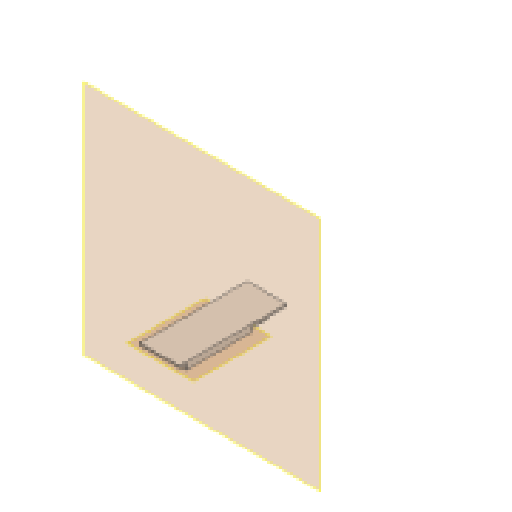
# Autodesk Inventor part: MCU seatbelt
Saved by Autodesk Inventor 2023 (Build 270158000, 158)
## iProperties
Created: 2025-01-03
Part Number: MCU seatbelt
Material: Generic
Document SubType Name: Modeling
Designer: jonwo
Density: 1 g/cm^3
Appearance: Default
Author: jonwo
Autodesk Inventor part; units mm, degrees
ref_plane "Work Plane1" through (0, 0, 0) normal (0, 0, 1) x (1, 0, 0)
sketch "Sketch1" plane through (0, 0, 0) normal (0, 0, 1) x (1, 0, 0)
  line L0 (-18.6403, -24.384) -> (-6.5903, -24.384) projected
  line L1 (-6.5903, -24.384) -> (-6.5903, -23.384) projected
  line L2 (-6.5903, -23.384) -> (-18.6403, -23.384) projected
  line L3 (-18.6403, -23.384) -> (-18.6403, -24.384) projected
  line L4 (-18.4403, -23.584) -> (-6.7903, -23.584)
  line L5 (-6.7903, -23.584) -> (-6.7903, -24.184)
  line L6 (-6.7903, -24.184) -> (-18.4403, -24.184)
  line L7 (-18.4403, -24.184) -> (-18.4403, -23.584)
  point P0 (0, 0)
  dimension "d0" = 0.2
  constraints: 8 end point, 3 other
  measures "d0" distance between parallel lines of L2 L4
ref_plane "Work Plane2" through (-20.1778, -24.509, -31.7) normal (0, 0, -1) x (0, 1, 0)
extrude "Extrusion1" add sketch "Sketch1" against normal up to surface (31.7 mm away) contours L4 L5 L6 L7
sketch "Sketch2" plane through (-18.4403, -24.184, 0) normal (0, -1, 0) x (1, 0, 0)
  line L0 (12.815, -1.2) -> (-1.155, -1.2) projected
  line L1 (-1.155, -22.155) -> (12.815, -22.155) projected
  line L2 (12.815, -2) -> (-1.155, -2)
  line L3 (-1.155, -21.355) -> (12.815, -21.355)
  line L4 (0, 0) -> (0, -31.7) projected
  line L5 (11.65, 0) -> (11.65, -31.7) projected
  point P0 (18.4403, 0)
  point P1 (11.65, -21.355)
  point P2 (11.65, -2)
  point P3 (0, -2)
  point P4 (0, -21.355)
  dimension "d3" = 0.8
  dimension "d4" = 0.8
  constraints: 4 end point, 2 parallel
  measures "d3" distance between parallel lines of L0 L2
  measures "d4" distance between parallel lines of L1 L3
ref_plane "Work Plane3" through (-12.6103, -25.6952, -11.6775) normal (0, 1, 0) x (0, 0, 1)
extrude "Extrusion2" add sketch "Sketch2" along normal up to surface (1.5112 mm away) contours L5 L3 L4 L2
sketch "Sketch3" plane through (-6.7903, -24.184, -21.355) normal (0, 0, -1) x (-1, 0, 0)
  line L0 (0, 0) -> (11.65, 0) projected
  line L1 (11.65, -1.5112) -> (0, -1.5112) projected
  line L2 (1, 0) -> (10.65, 0)
  line L3 (10.65, 0) -> (10.65, -1.5112)
  line L4 (10.65, -1.5112) -> (1, -1.5112)
  line L5 (1, -1.5112) -> (1, 0)
  line L6 (-1.05, -0.2) -> (2.45, -3.7) projected
  line L7 (8.7, -4.2) -> (12.7, -0.2) projected
  line L8 (0, 0) -> (0, -1.5112) projected
  line L9 (11.65, 0) -> (11.65, -1.5112) projected
  point P0 (-6.7903, 24.184)
  point P1 (1, -1.5112)
  dimension "d7" = 1
  dimension "d8" = 1
  constraints: 8 end point, 2 parallel, 2 point on line, 1 horizontal, 1 perpendicular
  measures "d7" distance between parallel lines of L8 L5
  measures "d8" distance between parallel lines of L9 L3
ref_plane "Work Plane4" through (-15.4903, -24.384, -27.0904) normal (0, 0, 1) x (1, 0, 0)
extrude "Extrusion3" add sketch "Sketch3" along normal up to surface (5.7354 mm away) contours L0 L3 L1 L5
sketch "Sketch4" plane through (-18.4403, -25.6952, -2) normal (0, -1, 0) x (1, 0, 0)
  line L0 (0, 2) -> (0, -29.7) projected
  line L1 (11.65, 2) -> (11.65, -29.7) projected
  line L2 (0, -14.85) -> (11.65, -14.85)
  line L3 (11.65, -14.85) -> (11.65, -13.85)
  line L4 (11.65, -13.85) -> (0, -13.85)
  line L5 (0, -13.85) -> (0, -14.85)
  line L6 (0, -5.2891) -> (11.65, -5.2891)
  line L7 (11.65, -5.2891) -> (11.65, -4.2891)
  line L8 (11.65, -4.2891) -> (0, -4.2891)
  line L9 (0, -4.2891) -> (0, -5.2891)
  point P0 (18.4403, 2)
  point P1 (0, -4.2891)
  point P2 (0, -5.2891)
  point P3 (0, -13.85)
  dimension "d11" = 1
  dimension "d12" = 1
  constraints: 16 end point, 4 parallel, 3 point on line, 2 horizontal, 2 perpendicular, 1 midpoint
  measures "d11" distance between parallel lines of L8 L6
  measures "d12" distance between parallel lines of L2 L4
ref_plane "Work Plane5" through (-21.5003, -26, -22.155) normal (0, 1, 0) x (0, 0, 1)
extrude "Extrusion4" [suppressed]
fillet "Fillet1" [suppressed]
equation "\"d8\" = d7"
equation "\"d12\" = d11"
body "Solid1"
